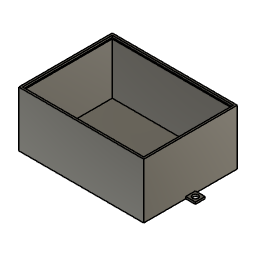
Tip rack holder v3 (Autodesk Fusion 360 design; units mm, degrees)
Autodesk Fusion 360 part; units mm, degrees
sketch "Sketch1" plane through (0, 0, 0) normal (0, 0, 1) x (1, 0, 0)
  line L0 (0, 0) -> (129, 0)
  line L1 (129, 0) -> (129, 96.5)
  line L2 (129, 96.5) -> (0, 96.5)
  line L3 (0, 96.5) -> (0, 0)
  line L4 (3.25, 3.25) -> (125.75, 3.25)
  line L5 (125.75, 3.25) -> (125.75, 93.25)
  line L6 (125.75, 93.25) -> (3.25, 93.25)
  line L7 (3.25, 93.25) -> (3.25, 3.25)
  dimension "d1" = 129
  dimension "d2" = 96.5
  dimension "d3" = 122.5
  dimension "d4" = 90
  dimension "d5" = 3.25
  dimension "d6" = 3.25
  constraint horizontal L0
  constraint vertical L1
  constraint horizontal L2
  constraint vertical L3
  constraint coincident L0.start L3.end
  constraint horizontal L4
  constraint vertical L5
  constraint horizontal L6
  constraint vertical L7
  measures "d1" distance of L0.start L0.end
  measures "d2" distance of L0.start L2.end
  measures "d3" distance of L4.start L4.end
  measures "d4" distance of L4.start L6.end
  measures "d5" distance of L3 L7
  measures "d6" distance of L0 L4
extrude "Extrude1" add sketch "Sketch1" along normal blind 5
sketch "Sketch2" plane through (0, 0, 5) normal (0, 0, 1) x (-1, 0, 0)
  line L0 (-3.25, -3.25) -> (-3.25, -93.25)
  line L1 (-3.25, -93.25) -> (-125.75, -93.25)
  line L2 (-125.75, -93.25) -> (-125.75, -3.25)
  line L3 (-125.75, -3.25) -> (-3.25, -3.25)
  line L4 (0, -96.5) -> (0, 0)
  line L5 (0, 0) -> (-129, 0)
  line L6 (-129, 0) -> (-129, -96.5)
  line L7 (-129, -96.5) -> (0, -96.5)
  line L8 (-2, -2) -> (-127, -2)
  line L9 (-127, -2) -> (-127, -94.5)
  line L10 (-127, -94.5) -> (-2, -94.5)
  line L11 (-2, -94.5) -> (-2, -2)
  dimension "d9" = 125
  dimension "d10" = 92.5
  dimension "d11" = 2
  dimension "d12" = 2
  constraint horizontal L8
  constraint vertical L9
  constraint horizontal L10
  constraint vertical L11
  measures "d9" distance of L8.start L8.end
  measures "d10" distance of L8.start L10.end
  measures "d11" distance of L5 L8
  measures "d12" distance of L4 L11
extrude "Extrude2" cut sketch "Sketch2" against normal blind 2 contours L8 L9 L10 L11
move_face "OffsetFaces1" offset 50 1 faces at (84.9167, 1.0833, 0)
sketch "Sketch4" plane through (129, 0, 0) normal (1, 0, 0) x (0, 1, 0)
  line L0 (0, -50) -> (96.5, -50)
  line L1 (96.5, -50) -> (96.5, 5)
  line L2 (96.5, 5) -> (0, 5)
  line L3 (0, 5) -> (0, -50)
  line L4 (0, -50) -> (96.5, -50)
  line L5 (96.5, -50) -> (96.5, -52)
  line L6 (96.5, -52) -> (0, -52)
  line L7 (0, -52) -> (0, -50)
  dimension "d18" = 96.5
  dimension "d19" = 2
  constraint horizontal L4
  constraint vertical L5
  constraint horizontal L6
  constraint vertical L7
  constraint coincident L0.start L3.end
  measures "d18" distance of L0.start L0.end
  measures "d19" distance of L0.start L6.end
extrude "Extrude3" add sketch "Sketch4" against normal blind 129 contours L0 L4 L5 L6 L7
sketch "Sketch5" plane through (129, 0, 0) normal (1, 0, 0) x (0, 1, 0)
  line L0 (96.5, -52) -> (96.5, 5)
  line L1 (96.5, 5) -> (0, 5)
  line L2 (0, 5) -> (0, -52)
  line L3 (0, -52) -> (96.5, -52)
  line L4 (43.25, -52) -> (53.25, -52)
  line L5 (53.25, -52) -> (53.25, -50)
  line L6 (53.25, -50) -> (43.25, -50)
  line L7 (43.25, -50) -> (43.25, -52)
  dimension "d22" = 10
  dimension "d23" = 2
  dimension "d24" = 43.25
  constraint horizontal L4
  constraint vertical L5
  constraint horizontal L6
  constraint vertical L7
  constraint coincident L3 L4.start
  measures "d22" distance of L4.start L4.end
  measures "d23" distance of L4.start L6.end
  measures "d24" distance of L2 L7
sketch "Sketch6" plane through (0, 0, 0) normal (-1, 0, 0) x (0, -1, 0)
  line L0 (0, -52) -> (0, 5)
  line L1 (0, 5) -> (-96.5, 5)
  line L2 (-96.5, 5) -> (-96.5, -52)
  line L3 (-96.5, -52) -> (0, -52)
  line L4 (-53.25, -52) -> (-43.25, -52)
  line L5 (-43.25, -52) -> (-43.25, -50)
  line L6 (-43.25, -50) -> (-53.25, -50)
  line L7 (-53.25, -50) -> (-53.25, -52)
  dimension "d25" = 10
  dimension "d26" = 2
  dimension "d27" = 43.25
  constraint horizontal L4
  constraint vertical L5
  constraint horizontal L6
  constraint vertical L7
  measures "d25" distance of L4.start L4.end
  measures "d26" distance of L4.start L6.end
  measures "d27" distance of L2 L7
extrude "Extrude4" add sketch "Sketch6" along normal blind 10 contours L3 L4 L5 L6 L7
extrude "Extrude5" add sketch "Sketch5" along normal blind 10 contours L3 L4 L5 L6 L7
sketch "Sketch7" plane through (0, 0, -50) normal (0, 0, 1) x (-1, 0, 0)
  line L0 (0, -43.25) -> (0, -53.25)
  line L1 (0, -53.25) -> (10, -53.25)
  line L2 (10, -53.25) -> (10, -43.25)
  line L3 (10, -43.25) -> (0, -43.25)
  circle A0 centre (5, -48.25) radius 3
  dimension "d32" = 6
  dimension "d33" = 5
  dimension "d34" = 5
  measures "d32" diameter of A0
  measures "d33" distance of L1 A0.centre
  measures "d34" distance of L2 A0.centre
extrude "Extrude6" cut sketch "Sketch7" against normal blind 2 contours A0
sketch "Sketch8" plane through (0, 0, -50) normal (0, 0, 1) x (-1, 0, 0)
  line L0 (-129, -53.25) -> (-129, -43.25)
  line L1 (-129, -43.25) -> (-139, -43.25)
  line L2 (-139, -43.25) -> (-139, -53.25)
  line L3 (-139, -53.25) -> (-129, -53.25)
  circle A0 centre (-134, -48.25) radius 3
  dimension "d37" = 6
  dimension "d38" = 5
  dimension "d39" = 5
  measures "d37" diameter of A0
  measures "d38" distance of L3 A0.centre
  measures "d39" distance of L2 A0.centre
extrude "Extrude7" cut sketch "Sketch8" against normal blind 2 contours A0
